# Autodesk Inventor part: ISOLATED_CON_2X04
Saved by Autodesk Inventor 2016 (Build 200138000, 138)
## iProperties
Created: 2016-04-08
Part Number: ISOLATED_CON_2X04
Material: Generic
Document SubType Name: Modeling
Designer: Paschalis
Density: 1 g/cm^3
Appearance: 2X04, ISOLATED_CON_2X04
Author: Paschalis
Autodesk Inventor part; units mm, degrees
ref_plane "YZ Plane" through (0, 0, 0) normal (1, 0, 0) x (0, 1, 0)
ref_plane "XZ Plane" through (0, 0, 0) normal (0, 1, 0) x (-1, 0, 0)
ref_plane "XY Plane" through (0, 0, 0) normal (0, 0, 1) x (1, 0, 0)
sketch "2X04, ISOLATED_CON_2X04_67" plane through (0, 0, 0) normal (0, 0, 1) x (1, 0, 0)
  line L0 (-5.1562, 2.54) -> (5.08, 2.54)
  line L1 (5.08, 2.54) -> (5.08, -2.6162)
  line L2 (5.08, -2.6162) -> (-5.1562, -2.6162)
  line L3 (-5.1562, -2.6162) -> (-5.1562, 2.54)
  constraints: 8 end point
extrude "Extrusion1" add sketch "2X04, ISOLATED_CON_2X04_67" along normal blind 1
body "Solid1"
